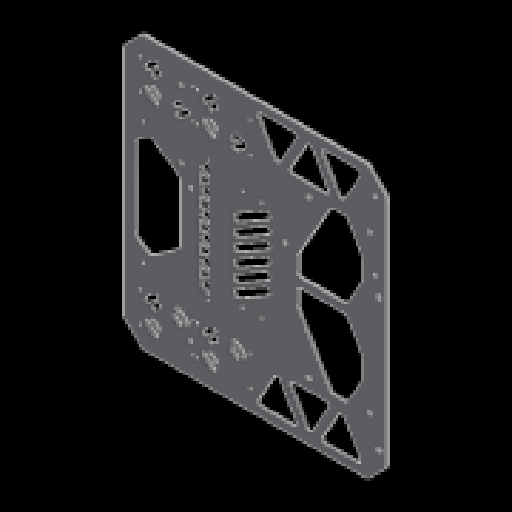
# Autodesk Inventor part: ChestTopPanel
Saved by Autodesk Inventor 2025.2 (Build 292293000, 293)
## iProperties
Created: 2025-10-05
Part Number: ChestTopPanel
Material: Generic
Document SubType Name: Sheet Metal
Designer: valer
Density: 1 g/cm^3
Sheet Metal Rule: Default
Appearance: Default
Author: valer
Autodesk Inventor part; units mm, degrees
ref_plane "YZ Plane" through (0, 0, 0) normal (1, 0, 0) x (0, 1, 0)
ref_plane "XZ Plane" through (0, 0, 0) normal (0, 1, 0) x (-1, 0, 0)
ref_plane "XY Plane" through (0, 0, 0) normal (0, 0, 1) x (1, 0, 0)
sketch "Base" plane through (0, 0, 0) normal (0, 0, 1) x (1, 0, 0)
  line L0 (370.5814, -180.975) -> (20.5814, -180.975)
  line L1 (20.5814, -180.975) -> (20.5814, 180.975)
  line L2 (20.5814, 180.975) -> (370.5814, 180.975)
  line L3 (370.5814, 180.975) -> (370.5814, -180.975)
  line L4 (-74.1163, 0) -> (444.6976, 0) construction
  point P0 (0, 0)
  point P1 (370.5814, 0)
  dimension "d1" = 361.95
  dimension "d3" = 350
  dimension "d55" = 20.5814
  measures "d1" distance of L2.end L0.start
  measures "d3" distance of L0.start L0.end
  measures "d55" distance from line of L1 point (0, 0)
extrude "Plate1" add sketch "Base" along normal blind 3
chamfer "BaseChamfersFeature" distance 25 angle 45 4 edges at (20.5814, 180.975, 1.5) (370.5814, 180.975, 1.5) (370.5814, -180.975, 1.5) (20.5814, -180.975, 1.5)
fillet "BaseFilletsFeature" radius 8 8 edges at (20.5814, 155.975, 1.5) (45.5814, 180.975, 1.5) (20.5814, -155.975, 1.5) (45.5814, -180.975, 1.5) (345.5814, 180.975, 1.5) (370.5814, 155.975, 1.5) (370.5814, -155.975, 1.5) (345.5814, -180.975, 1.5)
sketch "ChargerMountHoles" plane through (0, 0, 0) normal (0, 0, -1) x (-1, 0, 0)
  line L0 (-338.5814, 164.0145) -> (-338.5814, 43.4145) construction
  line L1 (-338.5814, 43.4145) -> (-358.8814, 43.4145) construction
  arc A0 (-364.5814, 49.1145) -> (-358.8814, 43.4145) centre (-358.8814, 49.1145) ccw construction
  line L2 (-364.5814, 49.1145) -> (-364.5814, 55.9145) construction
  line L3 (-364.5814, 55.9145) -> (-355.4314, 55.9145) construction
  arc A1 (-355.4314, 55.9145) -> (-355.4314, 61.6145) centre (-355.4314, 58.7645) ccw construction
  line L4 (-355.4314, 61.6145) -> (-364.5814, 61.6145) construction
  line L5 (-364.5814, 61.6145) -> (-364.5814, 145.8145) construction
  line L6 (-364.5814, 145.8145) -> (-355.4314, 145.8145) construction
  arc A2 (-355.4314, 145.8145) -> (-355.4314, 151.5145) centre (-355.4314, 148.6645) ccw construction
  line L7 (-355.4314, 151.5145) -> (-364.5814, 151.5145) construction
  line L8 (-364.5814, 151.5145) -> (-364.5814, 158.3145) construction
  arc A3 (-358.8814, 164.0145) -> (-364.5814, 158.3145) centre (-358.8814, 158.3145) ccw construction
  line L9 (-358.8814, 164.0145) -> (-338.5814, 164.0145) construction
  line L10 (-114.5814, 43.4145) -> (-114.5814, 164.0145) construction
  line L11 (-114.5814, 164.0145) -> (-94.2814, 164.0145) construction
  arc A4 (-88.5814, 158.3145) -> (-94.2814, 164.0145) centre (-94.2814, 158.3145) ccw construction
  line L12 (-88.5814, 158.3145) -> (-88.5814, 151.5145) construction
  line L13 (-88.5814, 151.5145) -> (-97.7314, 151.5145) construction
  arc A5 (-97.7314, 151.5145) -> (-97.7314, 145.8145) centre (-97.7314, 148.6645) ccw construction
  line L14 (-97.7314, 145.8145) -> (-88.5814, 145.8145) construction
  line L15 (-88.5814, 145.8145) -> (-88.5814, 61.6145) construction
  line L16 (-88.5814, 61.6145) -> (-97.7314, 61.6145) construction
  arc A6 (-97.7314, 61.6145) -> (-97.7314, 55.9145) centre (-97.7314, 58.7645) ccw construction
  line L17 (-97.7314, 55.9145) -> (-88.5814, 55.9145) construction
  line L18 (-88.5814, 55.9145) -> (-88.5814, 49.1145) construction
  arc A7 (-94.2814, 43.4145) -> (-88.5814, 49.1145) centre (-94.2814, 49.1145) ccw construction
  line L19 (-94.2814, 43.4145) -> (-114.5814, 43.4145) construction
  circle A8 centre (-97.7314, 58.7645) radius 2.5
  circle A9 centre (-97.7314, 148.6645) radius 2.5
  circle A10 centre (-355.4314, 58.7645) radius 2.5
  circle A11 centre (-355.4314, 148.6645) radius 2.5
  point P0 (0, 0)
  dimension "d14" = 5
  constraints: 4 centre point, 4 coincident, 3 equal radius
  measures "d14" diameter of A8
extrude "ChargerMountHolesFeature" cut sketch "ChargerMountHoles" against normal blind 3
sketch "ShelfMount" plane through (0, 0, 0) normal (0, 0, -1) x (-1, 0, 0)
  circle A0 centre (-360.5814, 36) radius 3
  circle A1 centre (-235.5814, 36) radius 3
  circle A2 centre (-110.5814, 36) radius 3
  circle A3 centre (-235.5814, 36) radius 3
  circle A4 centre (-110.5814, -140) radius 3
  circle A5 centre (-235.5814, -140) radius 3 construction
  circle A6 centre (-360.5814, -140) radius 3
  point P0 (0, 0)
  constraints: 7 centre point
extrude "ShelfMountFeature" cut sketch "ShelfMount" against normal blind 3
sketch "TopCuts" plane through (0, 0, 0) normal (0, 0, -1) x (-1, 0, 0)
  line L0 (-196.1462, 168.975) -> (-253.8813, 168.975)
  line L1 (-253.8813, 168.975) -> (-225.0138, 118.975)
  line L2 (-225.0138, 118.975) -> (-196.1462, 168.975)
  line L3 (-238.8702, 118.975) -> (-267.7377, 168.975)
  line L4 (-267.7377, 168.975) -> (-296.6052, 118.975)
  line L5 (-296.6052, 118.975) -> (-238.8702, 118.975)
  line L6 (-281.5941, 168.975) -> (-310.4616, 118.975)
  line L7 (-310.4616, 118.975) -> (-339.3291, 168.975)
  line L8 (-339.3291, 168.975) -> (-281.5941, 168.975)
  line L9 (-342.2676, 180.975) -> (-48.8951, 180.975) projected
  line L10 (-225.0138, 118.975) -> (-310.4616, 118.975) construction
  line L11 (-253.8813, 168.975) -> (-281.5941, 168.975) construction
  arc A0 (-342.2676, 180.975) -> (-347.9245, 178.6319) centre (-342.2676, 172.975) ccw projected
  line L12 (74.1163, 0) -> (-444.6976, 0) construction
  line L13 (-196.1462, -168.975) -> (-253.8813, -168.975)
  line L14 (-253.8813, -168.975) -> (-225.0138, -118.975)
  line L15 (-225.0138, -118.975) -> (-196.1462, -168.975)
  line L16 (-238.8702, -118.975) -> (-267.7377, -168.975)
  line L17 (-267.7377, -168.975) -> (-296.6052, -118.975)
  line L18 (-296.6052, -118.975) -> (-238.8702, -118.975)
  line L19 (-281.5941, -168.975) -> (-310.4616, -118.975)
  line L20 (-310.4616, -118.975) -> (-339.3291, -168.975)
  line L21 (-339.3291, -168.975) -> (-281.5941, -168.975)
  line L22 (-317.3898, 106.975) -> (-339.3291, 68.975)
  line L23 (-317.3898, 106.975) -> (-296.6052, 106.975)
  line L24 (-296.6052, 106.975) -> (-252.1637, 30)
  line L25 (-339.3291, 68.975) -> (-339.3291, 44.975)
  line L26 (-339.3291, 44.975) -> (-316.8269, 6)
  line L27 (-316.8269, 6) -> (-252.1637, 6)
  line L28 (-252.1637, 30) -> (-252.1637, 6)
  line L29 (-339.3291, 168.975) -> (-339.3291, 68.975) construction
  line L30 (-296.6052, 118.975) -> (-296.6052, 106.975) construction
  line L31 (-317.3898, -106.975) -> (-339.3291, -68.975)
  line L32 (-317.3898, -106.975) -> (-296.6052, -106.975)
  line L33 (-296.6052, -106.975) -> (-252.1637, -30)
  line L34 (-339.3291, -68.975) -> (-339.3291, -44.975)
  line L35 (-339.3291, -44.975) -> (-316.8269, -6)
  line L36 (-316.8269, -6) -> (-252.1637, -6)
  line L37 (-252.1637, -30) -> (-252.1637, -6)
  point P0 (0, 0)
  point P1 (-345.3291, 180.366)
  dimension "d39" = 60
  dimension "d40" = 60
  dimension "d41" = 60
  dimension "d42" = 60
  dimension "d43" = 12
  dimension "d44" = 12
  dimension "d45" = 6
  dimension "d46" = 62
  dimension "d47" = 12
  dimension "d48" = 120
  dimension "d49" = 24
  dimension "d50" = 24
  dimension "d51" = 6
  constraints: 74 end point, 16 symmetric about line, 5 parallel, 3 collinear, 3 horizontal, 3 perpendicular, 3 point on line, 1 midpoint, 1 point on circle, 1 vertical
  measures "d39" angle of L0 L2
  measures "d40" angle of L1 L0
  measures "d41" angle of L6 L8
  measures "d42" angle of L7 L8
  measures "d43" distance between parallel lines of L3 L1
  measures "d44" distance between parallel lines of L9 L0
  measures "d45" horizontal distance of point (-345.329, 180.366) L7.end
  measures "d46" distance between parallel lines of L9 L10
  measures "d47" distance between parallel lines of L23 L5
  measures "d48" angle of L24 L23
  measures "d49" distance of L22.end L25.end
  measures "d50" distance of L24.end L27.end
  measures "d51" distance between parallel lines of L12 L27
extrude "TopCutsFeature" cut sketch "TopCuts" against normal blind 3
fillet "TopCutFilletsFeature" radius 4 31 edges at (196.1462, 168.975, 1.5) (253.8813, 168.975, 1.5) (225.0138, 118.975, 1.5) (238.8702, 118.975, 1.5) (267.7377, 168.975, 1.5) (296.6052, 118.975, 1.5) (281.5941, 168.975, 1.5) (310.4616, 118.975, 1.5) (339.3291, 168.975, 1.5) (296.6052, 106.975, 1.5) (317.3898, 106.975, 1.5) (252.1637, 30, 1.5) (252.1637, 6, 1.5) (316.8269, 6, 1.5) (339.3291, 68.975, 1.5) (316.8269, -6, 1.5) (252.1637, -6, 1.5) (252.1637, -30, 1.5) (339.3291, -44.975, 1.5) (339.3291, -68.975, 1.5) (317.3898, -106.975, 1.5) (296.6052, -106.975, 1.5) (310.4616, -118.975, 1.5) (339.3291, -168.975, 1.5) (281.5941, -168.975, 1.5) (267.7377, -168.975, 1.5) (296.6052, -118.975, 1.5) (238.8702, -118.975, 1.5) (225.0138, -118.975, 1.5) (196.1462, -168.975, 1.5) (253.8813, -168.975, 1.5)
sketch "ComputerMountHoles" plane through (0, 0, 0) normal (0, 0, -1) x (-1, 0, 0)
  arc A0 (-270.2879, 102.25) -> (-264.5748, 102.25) centre (-267.4314, 104) ccw construction
  arc A1 (-350.2879, 102.25) -> (-344.5748, 102.25) centre (-347.4314, 104) ccw construction
  arc A2 (-270.2879, -105.75) -> (-264.5748, -105.75) centre (-267.4314, -104) ccw construction
  arc A3 (-350.2879, -105.75) -> (-344.5748, -105.75) centre (-347.4314, -104) ccw construction
  circle A4 centre (-267.4314, 104) radius 2.75
  circle A5 centre (-347.4314, 104) radius 2.75
  circle A6 centre (-347.4314, -104) radius 2.75
  circle A7 centre (-267.4314, -104) radius 2.75
  point P0 (0, 0)
  dimension "d56" = 3.35
  dimension "d57" = 5.5
  dimension "d58" = 5.5
  dimension "d59" = 5.5
  dimension "d60" = 5.5
  constraints: 4 centre point, 4 coincident
  measures "d56" radius of A0
  measures "d57" diameter of A4
  measures "d58" diameter of A5
  measures "d59" diameter of A6
  measures "d60" diameter of A7
extrude "ComputerMountHolesFeature" cut sketch "ComputerMountHoles" against normal blind 3
sketch "UsbHubMountHoles" plane through (0, 0, 0) normal (0, 0, -1) x (-1, 0, 0)
  circle A0 centre (-179.2814, 66.75) radius 2.25 construction
  circle A1 centre (-204.2814, 66.75) radius 2.25 construction
  circle A2 centre (-179.2814, -66.75) radius 2.25 construction
  circle A3 centre (-204.2814, -66.75) radius 2.25 construction
  circle A4 centre (-179.2814, -66.75) radius 1.75
  circle A5 centre (-204.2814, -66.75) radius 1.75
  circle A6 centre (-179.2814, 66.75) radius 1.75
  circle A7 centre (-204.2814, 66.75) radius 1.75
  point P0 (0, 0)
  dimension "d63" = 4.5
  dimension "d64" = 3.5
  dimension "d65" = 3.5
  dimension "d66" = 3.5
  dimension "d67" = 3.5
  constraints: 4 centre point, 4 coincident
  measures "d63" diameter of A2
  measures "d64" diameter of A4
  measures "d65" diameter of A5
  measures "d66" diameter of A6
  measures "d67" diameter of A7
extrude "UsbHubMountHolesFeature" cut sketch "UsbHubMountHoles" against normal blind 3
sketch "MainBoardMountHoles" plane through (0, 0, 0) normal (0, 0, -1) x (-1, 0, 0)
  circle A0 centre (-47.4314, 80.875) radius 1.6 construction
  circle A1 centre (-133.5814, 80.875) radius 1.6 construction
  circle A2 centre (-47.4314, -80.875) radius 1.6 construction
  circle A3 centre (-133.5814, -80.875) radius 1.6 construction
  circle A4 centre (-47.4314, 80.875) radius 1.25
  circle A5 centre (-133.5814, 80.875) radius 1.25
  circle A6 centre (-133.5814, -80.875) radius 1.25
  circle A7 centre (-47.4314, -80.875) radius 1.25
  point P0 (0, 0)
  dimension "d70" = 3.2
  dimension "d71" = 2.5
  dimension "d72" = 2.5
  dimension "d73" = 2.5
  dimension "d74" = 2.5
  constraints: 4 centre point, 4 coincident
  measures "d70" diameter of A0
  measures "d71" diameter of A4
  measures "d72" diameter of A5
  measures "d73" diameter of A6
  measures "d74" diameter of A7
extrude "MainBoardMountHolesFeature" cut sketch "MainBoardMountHoles" against normal blind 3
sketch "UsbHubVents" plane through (0, 0, 0) normal (0, 0, -1) x (-1, 0, 0)
  line L0 (74.1163, 0) -> (-444.6976, 0) construction
  line L1 (-171.7814, 60) -> (-211.7814, 60) construction
  line L2 (-211.7814, 60) -> (-211.7814, -60) construction
  line L3 (-211.7814, -60) -> (-171.7814, -60) construction
  line L4 (-171.7814, -60) -> (-171.7814, 60) construction
  circle A0 centre (-179.2814, 66.75) radius 1.75 construction
  circle A1 centre (-204.2814, 66.75) radius 1.75 construction
  line L5 (-179.2814, 66.75) -> (-204.2814, 66.75) construction
  line L6 (-191.7814, 66.75) -> (-191.7814, 60) construction
  line L7 (-171.7814, 32.406) -> (-211.7814, 55.5) construction
  line L8 (-169.5314, 36.3031) -> (-209.5314, 59.3971)
  line L9 (-214.0314, 51.6029) -> (-174.0314, 28.5089)
  arc A2 (-174.0314, 28.5089) -> (-169.5314, 36.3031) centre (-171.7814, 32.406) ccw
  arc A3 (-209.5314, 59.3971) -> (-214.0314, 51.6029) centre (-211.7814, 55.5) ccw
  arc A4 (-174.0314, 11.0089) -> (-169.5314, 18.8031) centre (-171.7814, 14.906) ccw
  line L10 (-169.5314, 18.8031) -> (-209.5314, 41.8971)
  line L11 (-214.0314, 34.1029) -> (-174.0314, 11.0089)
  arc A5 (-209.5314, 41.8971) -> (-214.0314, 34.1029) centre (-211.7814, 38) ccw
  arc A6 (-174.0314, -6.4911) -> (-169.5314, 1.3031) centre (-171.7814, -2.594) ccw
  line L12 (-169.5314, 1.3031) -> (-209.5314, 24.3971)
  line L13 (-214.0314, 16.6029) -> (-174.0314, -6.4911)
  arc A7 (-209.5314, 24.3971) -> (-214.0314, 16.6029) centre (-211.7814, 20.5) ccw
  arc A8 (-174.0314, -23.9911) -> (-169.5314, -16.1969) centre (-171.7814, -20.094) ccw
  line L14 (-169.5314, -16.1969) -> (-209.5314, 6.8971)
  line L15 (-214.0314, -0.8971) -> (-174.0314, -23.9911)
  arc A9 (-209.5314, 6.8971) -> (-214.0314, -0.8971) centre (-211.7814, 3) ccw
  arc A10 (-174.0314, -41.4911) -> (-169.5314, -33.6969) centre (-171.7814, -37.594) ccw
  line L16 (-169.5314, -33.6969) -> (-209.5314, -10.6029)
  line L17 (-214.0314, -18.3971) -> (-174.0314, -41.4911)
  arc A11 (-209.5314, -10.6029) -> (-214.0314, -18.3971) centre (-211.7814, -14.5) ccw
  arc A12 (-174.0314, -58.9911) -> (-169.5314, -51.1969) centre (-171.7814, -55.094) ccw
  line L18 (-169.5314, -51.1969) -> (-209.5314, -28.1029)
  line L19 (-214.0314, -35.8971) -> (-174.0314, -58.9911)
  arc A13 (-209.5314, -28.1029) -> (-214.0314, -35.8971) centre (-211.7814, -32) ccw
  point P0 (0, 0)
  point P1 (-171.7814, 0)
  point P2 (-191.7814, 43.953)
  point P3 (-211.7814, 42.5)
  point P4 (-211.7814, 25)
  point P5 (-211.7814, 7.5)
  point P6 (-211.7814, -10)
  point P7 (-211.7814, -27.5)
  dimension "d77" = 40
  dimension "d78" = 120
  dimension "d79" = 4.5
  dimension "d80" = 60
  dimension "d83" = 17.5
  constraints: 40 end point, 30 point on circle, 12 centre point, 4 midpoint, 4 tangent, 3 parallel, 3 point on line, 2 horizontal, 2 perpendicular, 1 vertical, 55 other
  measures "d77" distance of L2.end L3.end
  measures "d78" distance of L3.end L1.start
  measures "d79" radius of A2
  measures "d80" angle of L2 L7
  measures "d83" distance of L7.start A4.centre
extrude "UsbHubVentsFeature" cut sketch "UsbHubVents" against normal blind 3
sketch "ArmPowerBoardHoles" plane through (0, 0, 0) normal (0, 0, -1) x (-1, 0, 0)
  circle A0 centre (-113.7916, 154.3949) radius 1.25 projected
  circle A1 centre (-119.7916, 153.9785) radius 1.25 projected
  circle A2 centre (-190.0018, 154.3949) radius 1.25 projected
  circle A3 centre (-190.0018, 113.8591) radius 1.25 projected
  circle A4 centre (-43.5814, 153.9785) radius 1.25 projected
  circle A5 centre (-43.5814, 114.2755) radius 1.25 projected
  circle A6 centre (-113.7916, 113.8591) radius 1.25 projected
  circle A7 centre (-119.7916, 114.2755) radius 1.25 projected
  line L0 (-444.6976, 0) -> (74.1163, 0) construction
  circle A8 centre (-113.7916, -154.3949) radius 1.25
  circle A9 centre (-119.7916, -153.9785) radius 1.25
  circle A10 centre (-190.0018, -154.3949) radius 1.25
  circle A11 centre (-190.0018, -113.8591) radius 1.25
  circle A12 centre (-43.5814, -153.9785) radius 1.25
  circle A13 centre (-43.5814, -114.2755) radius 1.25
  circle A14 centre (-113.7916, -113.8591) radius 1.25
  circle A15 centre (-119.7916, -114.2755) radius 1.25
  point P0 (0, 0)
  constraints: 8 centre point, 8 symmetric about line, 8 other
extrude "ArmPowerBoardHolesFeature" cut sketch "ArmPowerBoardHoles" against normal blind 3
sketch "ArmPowerBoardVents" plane through (0, 0, 0) normal (0, 0, -1) x (-1, 0, 0)
  arc A0 (-66.1051, 114.8391) -> (-64.2514, 109.1327) centre (-65.1783, 111.9859) ccw projected
  arc A1 (-66.1051, 114.8391) -> (-55.1982, 123.3955) centre (-72.3314, 134.0055) ccw projected
  arc A2 (-50.0971, 120.2366) -> (-55.1982, 123.3955) centre (-52.6477, 121.816) ccw projected
  arc A3 (-64.2514, 109.1327) -> (-50.0971, 120.2366) centre (-72.3314, 134.0055) ccw projected
  arc A4 (-91.8957, 153.2365) -> (-93.9133, 158.8871) centre (-92.9045, 156.0618) ccw projected
  arc A5 (-91.8957, 153.2365) -> (-102.2577, 144.9526) centre (-85.0416, 134.0402) ccw projected
  arc A6 (-107.3255, 148.1648) -> (-102.2577, 144.9526) centre (-104.7916, 146.5587) ccw projected
  arc A7 (-93.9133, 158.8871) -> (-107.3255, 148.1648) centre (-85.0416, 134.0402) ccw projected
  arc A8 (-69.0096, 124.0151) -> (-66.0859, 118.7756) centre (-67.5478, 121.3953) ccw projected
  arc A9 (-69.0096, 124.0151) -> (-63.5903, 128.4264) centre (-78.8293, 141.6131) ccw projected
  arc A10 (-59.0531, 124.5003) -> (-63.5903, 128.4264) centre (-61.3217, 126.4634) ccw projected
  arc A11 (-66.0859, 118.7756) -> (-59.0531, 124.5003) centre (-78.8293, 141.6131) ccw projected
  arc A12 (-63.5599, 139.5367) -> (-59.0014, 143.438) centre (-61.2806, 141.4874) ccw projected
  arc A13 (-63.5599, 139.5367) -> (-68.955, 143.9776) centre (-78.8708, 126.4336) ccw projected
  arc A14 (-66.0028, 149.2011) -> (-68.955, 143.9776) centre (-67.4789, 146.5893) ccw projected
  arc A15 (-59.0014, 143.438) -> (-66.0028, 149.2011) centre (-78.8708, 126.4336) ccw projected
  arc A16 (-88.4179, 143.9776) -> (-91.3701, 149.2011) centre (-89.894, 146.5893) ccw projected
  arc A17 (-88.4179, 143.9776) -> (-93.813, 139.5367) centre (-78.5021, 126.4336) ccw projected
  arc A18 (-98.3716, 143.438) -> (-93.813, 139.5367) centre (-96.0923, 141.4874) ccw projected
  arc A19 (-91.3701, 149.2011) -> (-98.3716, 143.438) centre (-78.5021, 126.4336) ccw projected
  arc A20 (-93.8429, 128.5918) -> (-98.4227, 124.7155) centre (-96.1328, 126.6536) ccw projected
  arc A21 (-93.8429, 128.5918) -> (-88.4722, 124.1215) centre (-78.4607, 141.6111) ccw projected
  arc A22 (-91.4529, 118.9142) -> (-88.4722, 124.1215) centre (-89.9625, 121.5178) ccw projected
  arc A23 (-98.4227, 124.7155) -> (-91.4529, 118.9142) centre (-78.4607, 141.6111) ccw projected
  arc A24 (-102.3171, 123.2221) -> (-107.4023, 120.0377) centre (-104.8597, 121.6299) ccw projected
  arc A25 (-102.3171, 123.2221) -> (-92.0005, 114.8817) centre (-85.0416, 134.0402) ccw projected
  arc A26 (-94.049, 109.2422) -> (-92.0005, 114.8817) centre (-93.0247, 112.062) ccw projected
  arc A27 (-107.4023, 120.0377) -> (-94.049, 109.2422) centre (-85.0416, 134.0402) ccw projected
  arc A28 (-55.1405, 144.5217) -> (-50.0222, 147.6527) centre (-52.5814, 146.0872) ccw projected
  arc A29 (-55.1405, 144.5217) -> (-66.0005, 153.1376) centre (-72.3314, 134.0055) ccw projected
  arc A30 (-64.1156, 158.8338) -> (-66.0005, 153.1376) centre (-65.058, 155.9857) ccw projected
  arc A31 (-50.0222, 147.6527) -> (-64.1156, 158.8338) centre (-72.3314, 134.0055) ccw projected
  circle A32 centre (-43.5814, 153.9785) radius 1.25 projected
  circle A33 centre (-113.7916, 113.8591) radius 1.25 projected
  circle A34 centre (-43.5814, 114.2755) radius 1.25 projected
  circle A35 centre (-113.7916, 154.3949) radius 1.25 projected
  line L0 (-78.0472, 177.3414) -> (-41.5814, 156.2879) projected
  arc A36 (-78.0472, 177.3414) -> (-80.0472, 177.3414) centre (-79.0472, 175.6094) ccw projected
  line L1 (-115.7916, 156.7044) -> (-80.0472, 177.3414) projected
  arc A37 (-115.7916, 156.7044) -> (-116.7916, 154.9723) centre (-114.7916, 154.9723) ccw projected
  line L2 (-116.7916, 113.2817) -> (-116.7916, 154.9723) projected
  arc A38 (-116.7916, 113.2817) -> (-115.7916, 111.5496) centre (-114.7916, 113.2817) ccw projected
  line L3 (-79.6865, 90.7044) -> (-115.7916, 111.5496) projected
  arc A39 (-79.6865, 90.7044) -> (-77.6865, 90.7044) centre (-78.6865, 92.4364) ccw projected
  line L4 (-41.5814, 111.5496) -> (-77.6865, 90.7044) projected
  arc A40 (-41.5814, 111.5496) -> (-40.5814, 113.2817) centre (-42.5814, 113.2817) ccw projected
  line L5 (-40.5814, 154.5558) -> (-40.5814, 113.2817) projected
  arc A41 (-40.5814, 154.5558) -> (-41.5814, 156.2879) centre (-42.5814, 154.5558) ccw projected
  arc A42 (-142.3154, 114.8391) -> (-140.4616, 109.1327) centre (-141.3885, 111.9859) ccw projected
  arc A43 (-142.3154, 114.8391) -> (-131.4085, 123.3955) centre (-148.5416, 134.0055) ccw projected
  arc A44 (-126.3074, 120.2366) -> (-131.4085, 123.3955) centre (-128.8579, 121.816) ccw projected
  arc A45 (-140.4616, 109.1327) -> (-126.3074, 120.2366) centre (-148.5416, 134.0055) ccw projected
  arc A46 (-168.106, 153.2365) -> (-170.1235, 158.8871) centre (-169.1147, 156.0618) ccw projected
  arc A47 (-168.106, 153.2365) -> (-178.468, 144.9526) centre (-161.2518, 134.0402) ccw projected
  arc A48 (-183.5357, 148.1648) -> (-178.468, 144.9526) centre (-181.0018, 146.5587) ccw projected
  arc A49 (-170.1235, 158.8871) -> (-183.5357, 148.1648) centre (-161.2518, 134.0402) ccw projected
  arc A50 (-145.2198, 124.0151) -> (-142.2962, 118.7756) centre (-143.758, 121.3953) ccw projected
  arc A51 (-145.2198, 124.0151) -> (-139.8005, 128.4264) centre (-155.0396, 141.6131) ccw projected
  arc A52 (-135.2633, 124.5003) -> (-139.8005, 128.4264) centre (-137.5319, 126.4634) ccw projected
  arc A53 (-142.2962, 118.7756) -> (-135.2633, 124.5003) centre (-155.0396, 141.6131) ccw projected
  arc A54 (-139.7701, 139.5367) -> (-135.2116, 143.438) centre (-137.4909, 141.4874) ccw projected
  arc A55 (-139.7701, 139.5367) -> (-145.1653, 143.9776) centre (-155.081, 126.4336) ccw projected
  arc A56 (-142.213, 149.2011) -> (-145.1653, 143.9776) centre (-143.6892, 146.5893) ccw projected
  arc A57 (-135.2116, 143.438) -> (-142.213, 149.2011) centre (-155.081, 126.4336) ccw projected
  arc A58 (-164.6281, 143.9776) -> (-167.5804, 149.2011) centre (-166.1043, 146.5893) ccw projected
  arc A59 (-164.6281, 143.9776) -> (-170.0233, 139.5367) centre (-154.7124, 126.4336) ccw projected
  arc A60 (-174.5818, 143.438) -> (-170.0233, 139.5367) centre (-172.3025, 141.4874) ccw projected
  arc A61 (-167.5804, 149.2011) -> (-174.5818, 143.438) centre (-154.7124, 126.4336) ccw projected
  arc A62 (-170.0532, 128.5918) -> (-174.633, 124.7155) centre (-172.3431, 126.6536) ccw projected
  arc A63 (-170.0532, 128.5918) -> (-164.6824, 124.1215) centre (-154.6709, 141.6111) ccw projected
  arc A64 (-167.6631, 118.9142) -> (-164.6824, 124.1215) centre (-166.1728, 121.5178) ccw projected
  arc A65 (-174.633, 124.7155) -> (-167.6631, 118.9142) centre (-154.6709, 141.6111) ccw projected
  arc A66 (-178.5273, 123.2221) -> (-183.6126, 120.0377) centre (-181.0699, 121.6299) ccw projected
  arc A67 (-178.5273, 123.2221) -> (-168.2108, 114.8817) centre (-161.2518, 134.0402) ccw projected
  arc A68 (-170.2592, 109.2422) -> (-168.2108, 114.8817) centre (-169.235, 112.062) ccw projected
  arc A69 (-183.6126, 120.0377) -> (-170.2592, 109.2422) centre (-161.2518, 134.0402) ccw projected
  arc A70 (-131.3507, 144.5217) -> (-126.2325, 147.6527) centre (-128.7916, 146.0872) ccw projected
  arc A71 (-131.3507, 144.5217) -> (-142.2107, 153.1376) centre (-148.5416, 134.0055) ccw projected
  arc A72 (-140.3258, 158.8338) -> (-142.2107, 153.1376) centre (-141.2683, 155.9857) ccw projected
  arc A73 (-126.2325, 147.6527) -> (-140.3258, 158.8338) centre (-148.5416, 134.0055) ccw projected
  circle A74 centre (-119.7916, 153.9785) radius 1.25 projected
  circle A75 centre (-190.0018, 113.8591) radius 1.25 projected
  circle A76 centre (-119.7916, 114.2755) radius 1.25 projected
  circle A77 centre (-190.0018, 154.3949) radius 1.25 projected
  line L6 (-154.2574, 177.3414) -> (-117.7916, 156.2879) projected
  arc A78 (-154.2574, 177.3414) -> (-156.2574, 177.3414) centre (-155.2574, 175.6094) ccw projected
  line L7 (-192.0018, 156.7044) -> (-156.2574, 177.3414) projected
  arc A79 (-192.0018, 156.7044) -> (-193.0018, 154.9723) centre (-191.0018, 154.9723) ccw projected
  line L8 (-193.0018, 113.2817) -> (-193.0018, 154.9723) projected
  arc A80 (-193.0018, 113.2817) -> (-192.0018, 111.5496) centre (-191.0018, 113.2817) ccw projected
  line L9 (-155.8967, 90.7044) -> (-192.0018, 111.5496) projected
  arc A81 (-155.8967, 90.7044) -> (-153.8967, 90.7044) centre (-154.8967, 92.4364) ccw projected
  line L10 (-117.7916, 111.5496) -> (-153.8967, 90.7044) projected
  arc A82 (-117.7916, 111.5496) -> (-116.7916, 113.2817) centre (-118.7916, 113.2817) ccw projected
  line L11 (-116.7916, 154.5558) -> (-116.7916, 113.2817) projected
  arc A83 (-116.7916, 154.5558) -> (-117.7916, 156.2879) centre (-118.7916, 154.5558) ccw projected
  line L12 (74.1163, 0) -> (-444.6976, 0) construction
  arc A84 (-64.2514, -109.1327) -> (-66.1051, -114.8391) centre (-65.1783, -111.9859) ccw
  arc A85 (-55.1982, -123.3955) -> (-66.1051, -114.8391) centre (-72.3314, -134.0055) ccw
  arc A86 (-55.1982, -123.3955) -> (-50.0971, -120.2366) centre (-52.6477, -121.816) ccw
  arc A87 (-50.0971, -120.2366) -> (-64.2514, -109.1327) centre (-72.3314, -134.0055) ccw
  arc A88 (-93.9133, -158.8871) -> (-91.8957, -153.2365) centre (-92.9045, -156.0618) ccw
  arc A89 (-102.2577, -144.9526) -> (-91.8957, -153.2365) centre (-85.0416, -134.0402) ccw
  arc A90 (-102.2577, -144.9526) -> (-107.3255, -148.1648) centre (-104.7916, -146.5587) ccw
  arc A91 (-107.3255, -148.1648) -> (-93.9133, -158.8871) centre (-85.0416, -134.0402) ccw
  arc A92 (-66.0859, -118.7756) -> (-69.0096, -124.0151) centre (-67.5478, -121.3953) ccw
  arc A93 (-63.5903, -128.4264) -> (-69.0096, -124.0151) centre (-78.8293, -141.6131) ccw
  arc A94 (-63.5903, -128.4264) -> (-59.0531, -124.5003) centre (-61.3217, -126.4634) ccw
  arc A95 (-59.0531, -124.5003) -> (-66.0859, -118.7756) centre (-78.8293, -141.6131) ccw
  arc A96 (-59.0014, -143.438) -> (-63.5599, -139.5367) centre (-61.2806, -141.4874) ccw
  arc A97 (-68.955, -143.9776) -> (-63.5599, -139.5367) centre (-78.8708, -126.4336) ccw
  arc A98 (-68.955, -143.9776) -> (-66.0028, -149.2011) centre (-67.4789, -146.5893) ccw
  arc A99 (-66.0028, -149.2011) -> (-59.0014, -143.438) centre (-78.8708, -126.4336) ccw
  arc A100 (-91.3701, -149.2011) -> (-88.4179, -143.9776) centre (-89.894, -146.5893) ccw
  arc A101 (-93.813, -139.5367) -> (-88.4179, -143.9776) centre (-78.5021, -126.4336) ccw
  arc A102 (-93.813, -139.5367) -> (-98.3716, -143.438) centre (-96.0923, -141.4874) ccw
  arc A103 (-98.3716, -143.438) -> (-91.3701, -149.2011) centre (-78.5021, -126.4336) ccw
  arc A104 (-98.4227, -124.7155) -> (-93.8429, -128.5918) centre (-96.1328, -126.6536) ccw
  arc A105 (-88.4722, -124.1215) -> (-93.8429, -128.5918) centre (-78.4607, -141.6111) ccw
  arc A106 (-88.4722, -124.1215) -> (-91.4529, -118.9142) centre (-89.9625, -121.5178) ccw
  arc A107 (-91.4529, -118.9142) -> (-98.4227, -124.7155) centre (-78.4607, -141.6111) ccw
  arc A108 (-107.4023, -120.0377) -> (-102.3171, -123.2221) centre (-104.8597, -121.6299) ccw
  arc A109 (-92.0005, -114.8817) -> (-102.3171, -123.2221) centre (-85.0416, -134.0402) ccw
  arc A110 (-92.0005, -114.8817) -> (-94.049, -109.2422) centre (-93.0247, -112.062) ccw
  arc A111 (-94.049, -109.2422) -> (-107.4023, -120.0377) centre (-85.0416, -134.0402) ccw
  arc A112 (-50.0222, -147.6527) -> (-55.1405, -144.5217) centre (-52.5814, -146.0872) ccw
  arc A113 (-66.0005, -153.1376) -> (-55.1405, -144.5217) centre (-72.3314, -134.0055) ccw
  arc A114 (-66.0005, -153.1376) -> (-64.1156, -158.8338) centre (-65.058, -155.9857) ccw
  arc A115 (-64.1156, -158.8338) -> (-50.0222, -147.6527) centre (-72.3314, -134.0055) ccw
  arc A116 (-140.4616, -109.1327) -> (-142.3154, -114.8391) centre (-141.3885, -111.9859) ccw
  arc A117 (-131.4085, -123.3955) -> (-142.3154, -114.8391) centre (-148.5416, -134.0055) ccw
  arc A118 (-131.4085, -123.3955) -> (-126.3074, -120.2366) centre (-128.8579, -121.816) ccw
  arc A119 (-126.3074, -120.2366) -> (-140.4616, -109.1327) centre (-148.5416, -134.0055) ccw
  arc A120 (-170.1235, -158.8871) -> (-168.106, -153.2365) centre (-169.1147, -156.0618) ccw
  arc A121 (-178.468, -144.9526) -> (-168.106, -153.2365) centre (-161.2518, -134.0402) ccw
  arc A122 (-178.468, -144.9526) -> (-183.5357, -148.1648) centre (-181.0018, -146.5587) ccw
  arc A123 (-183.5357, -148.1648) -> (-170.1235, -158.8871) centre (-161.2518, -134.0402) ccw
  arc A124 (-142.2962, -118.7756) -> (-145.2198, -124.0151) centre (-143.758, -121.3953) ccw
  arc A125 (-139.8005, -128.4264) -> (-145.2198, -124.0151) centre (-155.0396, -141.6131) ccw
  arc A126 (-139.8005, -128.4264) -> (-135.2633, -124.5003) centre (-137.5319, -126.4634) ccw
  arc A127 (-135.2633, -124.5003) -> (-142.2962, -118.7756) centre (-155.0396, -141.6131) ccw
  arc A128 (-135.2116, -143.438) -> (-139.7701, -139.5367) centre (-137.4909, -141.4874) ccw
  arc A129 (-145.1653, -143.9776) -> (-139.7701, -139.5367) centre (-155.081, -126.4336) ccw
  arc A130 (-145.1653, -143.9776) -> (-142.213, -149.2011) centre (-143.6892, -146.5893) ccw
  arc A131 (-142.213, -149.2011) -> (-135.2116, -143.438) centre (-155.081, -126.4336) ccw
  arc A132 (-167.5804, -149.2011) -> (-164.6281, -143.9776) centre (-166.1043, -146.5893) ccw
  arc A133 (-170.0233, -139.5367) -> (-164.6281, -143.9776) centre (-154.7124, -126.4336) ccw
  arc A134 (-170.0233, -139.5367) -> (-174.5818, -143.438) centre (-172.3025, -141.4874) ccw
  arc A135 (-174.5818, -143.438) -> (-167.5804, -149.2011) centre (-154.7124, -126.4336) ccw
  arc A136 (-174.633, -124.7155) -> (-170.0532, -128.5918) centre (-172.3431, -126.6536) ccw
  arc A137 (-164.6824, -124.1215) -> (-170.0532, -128.5918) centre (-154.6709, -141.6111) ccw
  arc A138 (-164.6824, -124.1215) -> (-167.6631, -118.9142) centre (-166.1728, -121.5178) ccw
  arc A139 (-167.6631, -118.9142) -> (-174.633, -124.7155) centre (-154.6709, -141.6111) ccw
  arc A140 (-183.6126, -120.0377) -> (-178.5273, -123.2221) centre (-181.0699, -121.6299) ccw
  arc A141 (-168.2108, -114.8817) -> (-178.5273, -123.2221) centre (-161.2518, -134.0402) ccw
  arc A142 (-168.2108, -114.8817) -> (-170.2592, -109.2422) centre (-169.235, -112.062) ccw
  arc A143 (-170.2592, -109.2422) -> (-183.6126, -120.0377) centre (-161.2518, -134.0402) ccw
  arc A144 (-126.2325, -147.6527) -> (-131.3507, -144.5217) centre (-128.7916, -146.0872) ccw
  arc A145 (-142.2107, -153.1376) -> (-131.3507, -144.5217) centre (-148.5416, -134.0055) ccw
  arc A146 (-142.2107, -153.1376) -> (-140.3258, -158.8338) centre (-141.2683, -155.9857) ccw
  arc A147 (-140.3258, -158.8338) -> (-126.2325, -147.6527) centre (-148.5416, -134.0055) ccw
  point P0 (0, 0)
  constraints: 128 point on circle, 128 symmetric about line, 64 centre point, 64 other
extrude "ArmPowerBoardVentsFeature" cut sketch "ArmPowerBoardVents" against normal blind 3 contours A1 A2 A3 A0 | A9 A10 A11 A8 | A13 A14 A15 A12 | A21 A22 A23 A20 | A25 A26 A27 A24 | A29 A30 A31 A28 | A43 A44 A45 A42 | A51 A52 A53 A50 | A55 A56 A57 A54 | A63 A64 A65 A62 | A67 A68 A69 A66 | A71 A72 A73 A70 | A87 A86 A85 A84 | A95 A94 A93 A92 | A99 A98 A97 A96 | A107 A106 A105 A104 | A111 A110 A109 A108 | A115 A114 A113 A112 | A119 A118 A117 A116 | A127 A126 A125 A124 | A131 A130 A129 A128 | A139 A138 A137 A136 | A143 A142 A141 A140 | A147 A146 A145 A144
sketch "MainBoardVents" plane through (0, 0, 0) normal (0, 0, -1) x (-1, 0, 0)
  line L0 (-135.6814, 76.6856) -> (-135.6814, 58.2449)
  line L1 (-135.6814, 58.2449) -> (-122.5133, 67.4653)
  line L2 (-122.5133, 67.4653) -> (-135.6814, 76.6856)
  line L3 (-122.5133, 67.4653) -> (-135.6814, 67.4653) construction
  line L4 (-122.5133, 63.1926) -> (-135.6814, 53.9722)
  line L5 (-135.6814, 53.9722) -> (-122.5133, 44.7519)
  line L6 (-122.5133, 44.7519) -> (-122.5133, 63.1926)
  line L7 (-122.5133, 67.4653) -> (-122.5133, 63.1926) construction
  line L8 (-135.6814, 58.2449) -> (-135.6814, 53.9722) construction
  line L9 (-135.6814, 53.9722) -> (-122.5133, 53.9722) construction
  line L10 (-135.6814, 31.2588) -> (-135.6814, 49.6995)
  line L11 (-135.6814, 49.6995) -> (-122.5133, 40.4792)
  line L12 (-122.5133, 40.4792) -> (-135.6814, 31.2588)
  line L13 (-122.5133, 40.4792) -> (-135.6814, 40.4792) construction
  line L14 (-122.5133, 17.7658) -> (-135.6814, 26.9861)
  line L15 (-135.6814, 26.9861) -> (-122.5133, 36.2065)
  line L16 (-122.5133, 36.2065) -> (-122.5133, 17.7658)
  line L17 (-135.6814, 26.9861) -> (-122.5133, 26.9861) construction
  line L18 (-122.5133, 13.4931) -> (-135.6814, 22.7134)
  line L19 (-135.6814, 4.2727) -> (-122.5133, 13.4931)
  line L20 (-135.6814, 22.7134) -> (-135.6814, 4.2727)
  line L21 (-122.5133, 13.4931) -> (-135.6814, 13.4931) construction
  line L22 (-122.5133, -9.2203) -> (-122.5133, 9.2203)
  line L23 (-122.5133, 9.2203) -> (-135.6814, 0)
  line L24 (-135.6814, 0) -> (-122.5133, -9.2203)
  line L25 (74.1163, 0) -> (-444.6976, 0) construction
  line L26 (-135.6814, -76.6856) -> (-135.6814, -58.2449)
  line L27 (-135.6814, -58.2449) -> (-122.5133, -67.4653)
  line L28 (-122.5133, -67.4653) -> (-135.6814, -76.6856)
  line L29 (-122.5133, -63.1926) -> (-135.6814, -53.9722)
  line L30 (-135.6814, -53.9722) -> (-122.5133, -44.7519)
  line L31 (-122.5133, -44.7519) -> (-122.5133, -63.1926)
  line L32 (-122.5133, -40.4792) -> (-135.6814, -31.2588)
  line L33 (-135.6814, -49.6995) -> (-122.5133, -40.4792)
  line L34 (-135.6814, -31.2588) -> (-135.6814, -49.6995)
  line L35 (-122.5133, -36.2065) -> (-122.5133, -17.7658)
  line L36 (-122.5133, -17.7658) -> (-135.6814, -26.9861)
  line L37 (-135.6814, -26.9861) -> (-122.5133, -36.2065)
  line L38 (-135.6814, -4.2727) -> (-122.5133, -13.4931)
  line L39 (-122.5133, -13.4931) -> (-135.6814, -22.7134)
  line L40 (-135.6814, -22.7134) -> (-135.6814, -4.2727)
  point P0 (0, 0)
  point P1 (-141.6814, 81.025)
  point P2 (-135.6814, 87.025)
  point P3 (-122.5133, 0)
  dimension "d94" = 55
  dimension "d95" = 55
  dimension "d96" = 18.4407
  dimension "d97" = 6
  dimension "d98" = 55
  dimension "d99" = 55
  dimension "d100" = 3.5
  constraints: 80 end point, 27 symmetric about line, 6 midpoint, 2 equal length, 2 vertical, 1 collinear, 1 parallel, 1 point on line, 2 other
  measures "d94" angle of L0 L2
  measures "d95" angle of L1 L0
  measures "d96" distance of L0.start L0.end
  measures "d97" distance from line of L0 point (-141.681, 81.025)
  measures "d98" angle of L6 L4
  measures "d99" angle of L5 L6
  measures "d100" distance between parallel lines of L4 L1
extrude "MainBoardVentsFeature" cut sketch "MainBoardVents" against normal blind 3
fillet "MainBoardVentFilletsFeature" radius 2 33 edges at (122.5133, 67.4653, 1.5) (135.6814, 58.2449, 1.5) (135.6814, 76.6856, 1.5) (122.5133, 63.1926, 1.5) (135.6814, 53.9722, 1.5) (122.5133, 44.7519, 1.5) (122.5133, 40.4792, 1.5) (135.6814, 49.6995, 1.5) (135.6814, 31.2588, 1.5) (122.5133, 36.2065, 1.5) (122.5133, 17.7658, 1.5) (135.6814, 26.9861, 1.5) (135.6814, 22.7134, 1.5) (122.5133, 13.4931, 1.5) (135.6814, 4.2727, 1.5) (122.5133, 9.2203, 1.5) (135.6814, 0, 1.5) (122.5133, -9.2203, 1.5) (135.6814, -4.2727, 1.5) (122.5133, -13.4931, 1.5) (135.6814, -22.7134, 1.5) (122.5133, -17.7658, 1.5) (122.5133, -36.2065, 1.5) (135.6814, -26.9861, 1.5) (135.6814, -31.2588, 1.5) (122.5133, -40.4792, 1.5) (135.6814, -49.6995, 1.5) (122.5133, -44.7519, 1.5) (122.5133, -63.1926, 1.5) (135.6814, -53.9722, 1.5) (135.6814, -58.2449, 1.5) (122.5133, -67.4653, 1.5) (135.6814, -76.6856, 1.5)
sketch "WeightReliefCut2" plane through (0, 0, 0) normal (0, 0, -1) x (-1, 0, 0)
  line L0 (-56.5814, 69.0042) -> (-36.5814, 55)
  line L1 (-36.5814, 55) -> (-36.5814, -55)
  line L2 (-20.5814, 152.6613) -> (-20.5814, -152.6613) projected
  line L3 (-36.5814, -55) -> (-56.5814, -69.0042)
  line L4 (-56.5814, -69.0042) -> (-96.5814, -40.9958)
  line L5 (-96.5814, -40.9958) -> (-96.5814, 40.9958)
  line L6 (-96.5814, 40.9958) -> (-56.5814, 69.0042)
  line L7 (74.1163, 0) -> (-444.6976, 0) construction
  line L8 (-132.5342, 74.482) -> (-124.8531, 69.1036) projected
  line L9 (-124.8531, -69.1036) -> (-132.5342, -74.482) projected
  point P0 (0, 0)
  point P1 (-36.5814, 0)
  point P2 (-96.5814, 0)
  dimension "d104" = 16
  dimension "d105" = 60
  dimension "d106" = 20
  dimension "d107" = 110
  dimension "d108" = 110
  constraints: 12 end point, 4 parallel, 2 midpoint, 2 point on line, 1 equal length, 1 perpendicular
  measures "d104" distance between parallel lines of L2 L1
  measures "d105" distance between parallel lines of L1 L5
  measures "d106" horizontal distance of L0.start L0.end
  measures "d107" angle of L6 L0
  measures "d108" distance of L0.end L1.end
extrude "WeightReliefCut2Feature" cut sketch "WeightReliefCut2" against normal blind 3
fillet "WeightReliefCut2FilletsFeature" radius 6 6 edges at (36.5814, 55, 1.5) (56.5814, 69.0042, 1.5) (36.5814, -55, 1.5) (56.5814, -69.0042, 1.5) (96.5814, -40.9958, 1.5) (96.5814, 40.9958, 1.5)
equation "\"d15\" = Thickness"
equation "\"d29\" = Thickness"
equation "\"d52\" = Thickness"
equation "\"d4\" = Thickness"
equation "\"BendRadius\" = Thickness"
equation "\"BendReliefWidth\" = Thickness"
equation "\"BendReliefDepth\" = 0.5 * Thickness"
equation "\"CornerReliefSize\" = 4 * Thickness"
equation "\"MinimumRemnant\" = 2 * Thickness"
equation "\"TransitionRadius\" = BendRadius"
equation "\"JacobiRadiusSize\" = BendRadius"
equation "\"GapSize\" = Thickness"
equation "\"Thickness\" = 3"
body "Solid1"
